Autodesk Inventor part; units mm, degrees
(part 3 of 3)
  spline S438 degree 2 poles (-141.4024, 285.9166) (-141.5043, 285.3353) (-142.1656, 284.4468) (-142.8113, 284.1243) knots 0 0 0 1 2 2 2
  spline S439 degree 2 poles (-142.8113, 284.1243) (-142.9572, 284.0514) (-143.3044, 283.9167) (-143.468, 283.8902) knots 0 0 0 1 2 2 2
  line L516 (-143.468, 283.8902) -> (-143.8192, 284.5934)
  line L517 (-143.8192, 284.5934) -> (-143.7838, 284.611)
  spline S440 degree 2 poles (-143.7838, 284.611) (-143.6644, 284.6043) (-143.2289, 284.7059) (-143.0299, 284.8053) knots 0 0 0 1 2 2 2
  spline S441 degree 2 poles (-143.0299, 284.8053) (-142.3135, 285.1631) (-141.9681, 286.5182) (-142.348, 287.4225) knots 0 0 0 1 2 2 2
  spline S442 degree 2 poles (-142.348, 287.4225) (-142.5405, 287.0777) (-142.9806, 286.6313) (-143.2945, 286.4745) knots 0 0 0 1 2 2 2
  spline S443 degree 2 poles (-143.2945, 286.4745) (-143.5952, 286.3242) (-144.1612, 286.2073) (-144.5083, 286.2715) knots 0 0 0 1 2 2 2
  spline S444 degree 2 poles (-144.5083, 286.2715) (-144.9128, 286.3513) (-145.5559, 286.8865) (-145.7967, 287.3685) knots 0 0 0 1 2 2 2
  spline S445 degree 2 poles (-142.7655, 288.3025) (-143.0416, 288.8553) (-143.5941, 289.4524) (-143.8704, 289.552) knots 0 0 0 1 2 2 2
  spline S446 degree 2 poles (-143.8704, 289.552) (-144.1179, 289.6493) (-144.5159, 289.6163) (-144.7104, 289.5191) knots 0 0 0 1 2 2 2
  spline S447 degree 2 poles (-144.7104, 289.5191) (-145.1615, 289.2938) (-145.3741, 288.3809) (-145.0692, 287.7706) knots 0 0 0 1 2 2 2
  spline S448 degree 2 poles (-145.0692, 287.7706) (-144.8969, 287.4257) (-144.4969, 287.0674) (-144.2228, 287.0054) knots 0 0 0 1 2 2 2
  spline S449 degree 2 poles (-144.2228, 287.0054) (-144.0239, 286.9611) (-143.637, 287.0604) (-143.4335, 287.162) knots 0 0 0 1 2 2 2
  spline S450 degree 2 poles (-143.4335, 287.162) (-143.1992, 287.2791) (-142.7414, 287.7122) (-142.6064, 287.9509) knots 0 0 0 1 2 2 2
  spline S451 degree 2 poles (-142.6064, 287.9509) (-142.6285, 288.0062) (-142.7103, 288.192) (-142.7655, 288.3025) knots 0 0 0 1 2 2 2
  line L518 (-359.0969, 1.8042) -> (-364.0351, 1.8396)
  line L519 (-364.0351, 1.8396) -> (-364.048, 0.0353)
  line L520 (-364.048, 0.0353) -> (-365.2097, 0.0437)
  line L521 (-365.2097, 0.0437) -> (-365.1729, 5.1845)
  line L522 (-365.1729, 5.1845) -> (-364.0112, 5.1762)
  line L523 (-364.0112, 5.1762) -> (-364.0242, 3.372)
  line L524 (-364.0242, 3.372) -> (-359.086, 3.3366)
  line L525 (-359.086, 3.3366) -> (-359.0969, 1.8042)
  line L526 (-358.9438, 10.9181) -> (-358.9795, 9.3861)
  line L527 (-358.9795, 9.3861) -> (-361.6827, 9.4489)
  line L528 (-361.6827, 9.4489) -> (-361.7311, 7.3684)
  line L529 (-361.7311, 7.3684) -> (-359.0278, 7.3055)
  line L530 (-359.0278, 7.3055) -> (-359.0634, 5.7735)
  line L531 (-359.0634, 5.7735) -> (-365.1618, 5.9153)
  line L532 (-365.1618, 5.9153) -> (-365.1262, 7.4473)
  line L533 (-365.1262, 7.4473) -> (-362.8924, 7.3954)
  line L534 (-362.8924, 7.3954) -> (-362.8441, 9.4759)
  line L535 (-362.8441, 9.4759) -> (-365.0778, 9.5278)
  line L536 (-365.0778, 9.5278) -> (-365.0422, 11.0598)
  line L537 (-365.0422, 11.0598) -> (-358.9438, 10.9181)
  line L538 (-358.8992, 12.1827) -> (-364.9945, 12.4227)
  line L539 (-364.9945, 12.4227) -> (-364.8323, 16.5422)
  line L540 (-364.8323, 16.5422) -> (-363.6715, 16.4965)
  line L541 (-363.6715, 16.4965) -> (-363.7738, 13.8984)
  line L542 (-363.7738, 13.8984) -> (-362.702, 13.8562)
  line L543 (-362.702, 13.8562) -> (-362.6076, 16.2518)
  line L544 (-362.6076, 16.2518) -> (-361.4469, 16.2061)
  line L545 (-361.4469, 16.2061) -> (-361.5412, 13.8105)
  line L546 (-361.5412, 13.8105) -> (-360.0001, 13.7498)
  line L547 (-360.0001, 13.7498) -> (-359.8978, 16.3479)
  line L548 (-359.8978, 16.3479) -> (-358.737, 16.3022)
  line L549 (-358.737, 16.3022) -> (-358.8992, 12.1827)
  line L550 (-358.1711, 26.0089) -> (-358.2682, 24.4895)
  line L551 (-358.2682, 24.4895) -> (-362.3035, 24.7473)
  line L552 (-362.3035, 24.7473) -> (-359.7694, 23.4759)
  line L553 (-359.7694, 23.4759) -> (-359.8362, 22.43)
  line L554 (-359.8362, 22.43) -> (-362.5116, 21.4914)
  line L555 (-362.5116, 21.4914) -> (-358.4762, 21.2335)
  line L556 (-358.4762, 21.2335) -> (-358.5683, 19.7931)
  line L557 (-358.5683, 19.7931) -> (-364.6558, 20.1821)
  line L558 (-364.6558, 20.1821) -> (-364.5433, 21.9432)
  line L559 (-364.5433, 21.9432) -> (-361.4526, 23.1029)
  line L560 (-361.4526, 23.1029) -> (-364.3712, 24.6368)
  line L561 (-364.3712, 24.6368) -> (-364.2586, 26.3979)
  line L562 (-364.2586, 26.3979) -> (-358.1711, 26.0089)
  line L563 (-358.069, 27.2702) -> (-364.1488, 27.7664)
  line L564 (-364.1488, 27.7664) -> (-363.8134, 31.8755)
  line L565 (-363.8134, 31.8755) -> (-362.6556, 31.781)
  line L566 (-362.6556, 31.781) -> (-362.8671, 29.1894)
  line L567 (-362.8671, 29.1894) -> (-361.798, 29.1022)
  line L568 (-361.798, 29.1022) -> (-361.6029, 31.4917)
  line L569 (-361.6029, 31.4917) -> (-360.4451, 31.3972)
  line L570 (-360.4451, 31.3972) -> (-360.6401, 29.0077)
  line L571 (-360.6401, 29.0077) -> (-359.1029, 28.8822)
  line L572 (-359.1029, 28.8822) -> (-358.8914, 31.4738)
  line L573 (-358.8914, 31.4738) -> (-357.7336, 31.3793)
  line L574 (-357.7336, 31.3793) -> (-358.069, 27.2702)
  spline S452 degree 2 poles (-357.2701, 35.0194) (-357.4024, 33.6515) (-359.2108, 32.2074) (-360.7065, 32.3521) knots 0 0 0 1 2 2 2
  spline S453 degree 2 poles (-360.7065, 32.3521) (-362.1482, 32.4915) (-363.7098, 34.2666) (-363.5775, 35.6344) knots 0 0 0 1 2 2 2
  spline S454 degree 2 poles (-363.5775, 35.6344) (-363.5427, 35.9936) (-363.4029, 36.5661) (-363.3084, 36.8251) knots 0 0 0 1 2 2 2
  spline S455 degree 2 poles (-363.3084, 36.8251) (-363.2244, 37.0256) (-362.9657, 37.4922) (-362.8722, 37.6372) knots 0 0 0 1 2 2 2
  line L575 (-362.8722, 37.6372) -> (-361.4257, 37.4972)
  line L576 (-361.4257, 37.4972) -> (-361.4404, 37.3447)
  spline S456 degree 2 poles (-361.4404, 37.3447) (-361.5498, 37.2411) (-361.8577, 36.9331) (-362.0061, 36.7339) knots 0 0 0 1 2 2 2
  spline S457 degree 2 poles (-362.0061, 36.7339) (-362.1594, 36.5352) (-362.3904, 36.046) (-362.4176, 35.7656) knots 0 0 0 1 2 2 2
  spline S458 degree 2 poles (-362.4176, 35.7656) (-362.4494, 35.4359) (-362.2956, 34.8698) (-362.0591, 34.5936) knots 0 0 0 1 2 2 2
  spline S459 degree 2 poles (-362.0591, 34.5936) (-361.8498, 34.3449) (-361.0857, 33.978) (-360.5493, 33.9261) knots 0 0 0 1 2 2 2
  spline S460 degree 2 poles (-360.5493, 33.9261) (-359.9835, 33.8714) (-359.182, 34.0968) (-358.922, 34.32) knots 0 0 0 1 2 2 2
  spline S461 degree 2 poles (-358.922, 34.32) (-358.6679, 34.5338) (-358.41, 35.0949) (-358.382, 35.3852) knots 0 0 0 1 2 2 2
  spline S462 degree 2 poles (-358.382, 35.3852) (-358.3529, 35.6853) (-358.5018, 36.251) (-358.6068, 36.4499) knots 0 0 0 1 2 2 2
  spline S463 degree 2 poles (-358.6068, 36.4499) (-358.7098, 36.6684) (-358.9406, 37.0036) (-359.033, 37.1268) knots 0 0 0 1 2 2 2
  line L577 (-359.033, 37.1268) -> (-359.0196, 37.2645)
  line L578 (-359.0196, 37.2645) -> (-357.5927, 37.1265)
  spline S464 degree 2 poles (-357.5927, 37.1265) (-357.5302, 36.9516) (-357.3757, 36.4947) (-357.3297, 36.2518) knots 0 0 0 1 2 2 2
  spline S465 degree 2 poles (-357.3297, 36.2518) (-357.2687, 35.9579) (-357.2282, 35.4524) (-357.2701, 35.0194) knots 0 0 0 1 2 2 2
  line L579 (-356.514, 43.1002) -> (-356.6871, 41.5776)
  line L580 (-356.6871, 41.5776) -> (-359.3737, 41.8829)
  line L581 (-359.3737, 41.8829) -> (-359.6087, 39.8151)
  line L582 (-359.6087, 39.8151) -> (-356.922, 39.5098)
  line L583 (-356.922, 39.5098) -> (-357.095, 37.9872)
  line L584 (-357.095, 37.9872) -> (-363.156, 38.6759)
  line L585 (-363.156, 38.6759) -> (-362.983, 40.1985)
  line L586 (-362.983, 40.1985) -> (-360.7629, 39.9462)
  line L587 (-360.7629, 39.9462) -> (-360.528, 42.014)
  line L588 (-360.528, 42.014) -> (-362.748, 42.2663)
  line L589 (-362.748, 42.2663) -> (-362.575, 43.7889)
  line L590 (-362.575, 43.7889) -> (-356.514, 43.1002)
  line L591 (-356.4432, 43.7041) -> (-362.2241, 46.5396)
  line L592 (-362.2241, 46.5396) -> (-362.0073, 48.1963)
  line L593 (-362.0073, 48.1963) -> (-355.6914, 49.4486)
  line L594 (-355.6914, 49.4486) -> (-355.896, 47.885)
  line L595 (-355.896, 47.885) -> (-357.1806, 47.6693)
  line L596 (-357.1806, 47.6693) -> (-357.4295, 45.7675)
  line L597 (-357.4295, 45.7675) -> (-356.2443, 45.2235)
  line L598 (-356.2443, 45.2235) -> (-356.4432, 43.7041)
  line L599 (-358.3221, 47.4797) -> (-360.4028, 47.1238)
  line L600 (-360.4028, 47.1238) -> (-358.4844, 46.2396)
  line L601 (-358.4844, 46.2396) -> (-358.3221, 47.4797)
  line L602 (-354.8318, 55.2679) -> (-355.0479, 53.8108)
  line L603 (-355.0479, 53.8108) -> (-359.5982, 52.1068)
  line L604 (-359.5982, 52.1068) -> (-355.393, 51.4832)
  line L605 (-355.393, 51.4832) -> (-355.5982, 50.0994)
  line L606 (-355.5982, 50.0994) -> (-361.6322, 50.9941)
  line L607 (-361.6322, 50.9941) -> (-361.3567, 52.8523)
  line L608 (-361.3567, 52.8523) -> (-357.6139, 54.2662)
  line L609 (-357.6139, 54.2662) -> (-361.071, 54.7788)
  line L610 (-361.071, 54.7788) -> (-360.8658, 56.1627)
  line L611 (-360.8658, 56.1627) -> (-354.8318, 55.2679)
  line L612 (-354.1428, 59.488) -> (-354.6718, 56.2485)
  line L613 (-354.6718, 56.2485) -> (-355.7207, 56.4198)
  line L614 (-355.7207, 56.4198) -> (-355.5797, 57.2833)
  line L615 (-355.5797, 57.2833) -> (-359.5021, 57.9238)
  line L616 (-359.5021, 57.9238) -> (-359.6431, 57.0603)
  line L617 (-359.6431, 57.0603) -> (-360.692, 57.2315)
  line L618 (-360.692, 57.2315) -> (-360.1631, 60.471)
  line L619 (-360.1631, 60.471) -> (-359.1142, 60.2997)
  line L620 (-359.1142, 60.2997) -> (-359.2552, 59.4362)
  line L621 (-359.2552, 59.4362) -> (-355.3327, 58.7957)
  line L622 (-355.3327, 58.7957) -> (-355.1917, 59.6592)
  line L623 (-355.1917, 59.6592) -> (-354.1428, 59.488)
  spline S466 degree 2 poles (-353.4, 63.0613) (-353.6397, 61.7081) (-355.5562, 60.4109) (-357.0359, 60.673) knots 0 0 0 1 2 2 2
  spline S467 degree 2 poles (-357.0359, 60.673) (-358.4621, 60.9256) (-359.879, 62.8182) (-359.6393, 64.1713) knots 0 0 0 1 2 2 2
  spline S468 degree 2 poles (-359.6393, 64.1713) (-359.5764, 64.5267) (-359.3919, 65.0864) (-359.2772, 65.3372) knots 0 0 0 1 2 2 2
  spline S469 degree 2 poles (-359.2772, 65.3372) (-359.1777, 65.5304) (-358.8831, 65.9752) (-358.7785, 66.1123) knots 0 0 0 1 2 2 2
  line L624 (-358.7785, 66.1123) -> (-357.3474, 65.8588)
  line L625 (-357.3474, 65.8588) -> (-357.3741, 65.7079)
  spline S470 degree 2 poles (-357.3741, 65.7079) (-357.4913, 65.6132) (-357.8225, 65.3305) (-357.9861, 65.1436) knots 0 0 0 1 2 2 2
  spline S471 degree 2 poles (-357.9861, 65.1436) (-358.1546, 64.9576) (-358.4235, 64.4881) (-358.4727, 64.2107) knots 0 0 0 1 2 2 2
  spline S472 degree 2 poles (-358.4727, 64.2107) (-358.5304, 63.8846) (-358.4217, 63.3081) (-358.2077, 63.0141) knots 0 0 0 1 2 2 2
  spline S473 degree 2 poles (-358.2077, 63.0141) (-358.0186, 62.7497) (-357.2858, 62.3237) (-356.7552, 62.2298) knots 0 0 0 1 2 2 2
  spline S474 degree 2 poles (-356.7552, 62.2298) (-356.1954, 62.1306) (-355.3786, 62.2922) (-355.1019, 62.4942) knots 0 0 0 1 2 2 2
  spline S475 degree 2 poles (-355.1019, 62.4942) (-354.8317, 62.6873) (-354.5304, 63.2263) (-354.4796, 63.5135) knots 0 0 0 1 2 2 2
  spline S476 degree 2 poles (-354.4796, 63.5135) (-354.427, 63.8104) (-354.5309, 64.3861) (-354.6198, 64.5926) knots 0 0 0 1 2 2 2
  spline S477 degree 2 poles (-354.6198, 64.5926) (-354.7053, 64.8186) (-354.9089, 65.1709) (-354.9913, 65.301) knots 0 0 0 1 2 2 2
  line L626 (-354.9913, 65.301) -> (-354.9672, 65.4373)
  line L627 (-354.9672, 65.4373) -> (-353.5556, 65.1873)
  spline S478 degree 2 poles (-353.5556, 65.1873) (-353.507, 65.008) (-353.3891, 64.5403) (-353.3623, 64.2946) knots 0 0 0 1 2 2 2
  spline S479 degree 2 poles (-353.3623, 64.2946) (-353.3247, 63.9967) (-353.3241, 63.4896) (-353.4, 63.0613) knots 0 0 0 1 2 2 2
  spline S480 degree 2 poles (-352.5248, 67.8341) (-352.6577, 67.1449) (-353.125, 66.1576) (-353.4052, 65.7485) knots 0 0 0 1 2 2 2
  line L628 (-353.4052, 65.7485) -> (-354.8323, 66.0237)
  line L629 (-354.8323, 66.0237) -> (-354.806, 66.1596)
  spline S481 degree 2 poles (-354.806, 66.1596) (-354.3355, 66.537) (-353.7142, 67.5399) (-353.616, 68.0495) knots 0 0 0 1 2 2 2
  spline S482 degree 2 poles (-353.616, 68.0495) (-353.5907, 68.1806) (-353.5675, 68.6141) (-353.6014, 68.7516) knots 0 0 0 1 2 2 2
  spline S483 degree 2 poles (-353.6014, 68.7516) (-353.6394, 68.92) (-353.8449, 69.1861) (-354.0439, 69.2245) knots 0 0 0 1 2 2 2
  spline S484 degree 2 poles (-354.0439, 69.2245) (-354.272, 69.2685) (-354.6218, 68.9685) (-354.7317, 68.7379) knots 0 0 0 1 2 2 2
  spline S485 degree 2 poles (-354.7317, 68.7379) (-354.8732, 68.4481) (-355.1478, 67.7811) (-355.3136, 67.4959) knots 0 0 0 1 2 2 2
  spline S486 degree 2 poles (-355.3136, 67.4959) (-355.6901, 66.8486) (-356.6362, 66.4068) (-357.2575, 66.5266) knots 0 0 0 1 2 2 2
  spline S487 degree 2 poles (-357.2575, 66.5266) (-358.0972, 66.6885) (-358.8665, 68.3119) (-358.6606, 69.3798) knots 0 0 0 1 2 2 2
  spline S488 degree 2 poles (-358.6606, 69.3798) (-358.5577, 69.9137) (-358.1352, 70.9297) (-357.8703, 71.3116) knots 0 0 0 1 2 2 2
  line L630 (-357.8703, 71.3116) -> (-356.5015, 71.0476)
  line L631 (-356.5015, 71.0476) -> (-356.5268, 70.9166)
  spline S489 degree 2 poles (-356.5268, 70.9166) (-356.8777, 70.6369) (-357.4562, 69.7516) (-357.5535, 69.2468) knots 0 0 0 1 2 2 2
  spline S490 degree 2 poles (-357.5535, 69.2468) (-357.5919, 69.0478) (-357.5936, 68.7259) (-357.5496, 68.5362) knots 0 0 0 1 2 2 2
  spline S491 degree 2 poles (-357.5496, 68.5362) (-357.5136, 68.3833) (-357.3006, 68.1308) (-357.1452, 68.1008) knots 0 0 0 1 2 2 2
  spline S492 degree 2 poles (-357.1452, 68.1008) (-356.9122, 68.0559) (-356.5826, 68.3296) (-356.3859, 68.775) knots 0 0 0 1 2 2 2
  spline S493 degree 2 poles (-356.3859, 68.775) (-356.2599, 69.0628) (-356.0213, 69.5957) (-355.8478, 69.8946) knots 0 0 0 1 2 2 2
  spline S494 degree 2 poles (-355.8478, 69.8946) (-355.4999, 70.4719) (-354.6257, 70.9326) (-354.0044, 70.8128) knots 0 0 0 1 2 2 2
  spline S495 degree 2 poles (-354.0044, 70.8128) (-353.1113, 70.6406) (-352.2945, 69.0281) (-352.5248, 67.8341) knots 0 0 0 1 2 2 2
  constraints: 2 centre point, 2 coincident, 2 other
extrude "Extrusion11" cut sketch "Sketch11" against normal blind 1 contours L320 L321 L322 S221 S222 S219 S220 | L0 L1 L2 S2 S3 S0 S1 | L510 L511 L512 L513 L514 L515 L509 | L6 L7 L8 L9 L10 L11 L12 L13 L14 L15 L16 L17 | L36 L25 L26 L27 L28 L29 L30 L31 L32 L33 L34 L35 | L103 L104 L105 L106 L107 L108 L109 L116 | L124 L125 L126 L127 L128 L129 L130 L131 L120 L121 L122 L123 | L150 L151 S119 S120 S121 S122 S123 S124 L152 L153 S125 S126 S127 S128 S129 L154 L155 | L156 L157 L158 L159 L160 L161 S130 L162 L163 L164 L165 | L168 L169 L170 S152 S153 S150 S151 | L250 L251 L252 L253 L254 L255 L256 L257 L258 L246 L247 L248 L249 | L352 L353 S281 S282 S283 S284 S285 S286 L354 L355 S287 S288 S289 S290 S291 L356 L357 | L399 L388 L389 L390 L391 L392 L393 L394 L395 L396 L397 L398 | L400 L401 L402 L403 L404 L405 | L433 L422 L423 L424 L425 L426 L427 L428 L429 L430 L431 L432 | L440 L441 L442 L443 L434 L435 L436 L437 L438 L439 | L477 L478 L479 S373 S374 S371 S372 | S379 L495 L496 S380 S381 S382 S383 S384 S385 S386 S387 L497 L498 S388 S389 S390 S391 S392 S393 S394 A1 | A1 S394 S379 | A1 L414 L415 L416 L417 L418 L419 L420 | S397 S398 S399 S400 S401 L499 L500 S402 S403 S404 S405 S406 S395 S396 A1 | A1 S396 S397 | S370 S355 A1 | A1 S355 L410 L411 S356 S357 S358 S359 S360 S361 S362 S363 L412 L413 S364 S365 S366 S367 S368 S369 S370 | S424 L504 L505 S425 S426 S427 S428 S429 L506 L507 L508 S430 S431 S432 S414 S415 L501 L502 S416 S417 S418 S419 L503 S420 S421 S422 S423 A1 | A1 S423 S424 | S354 S339 A1 | A1 S339 L406 L407 S340 S341 S342 S343 S344 S345 S346 S347 L408 L409 S348 S349 S350 S351 S352 S353 S354 | L516 L517 S440 S441 S442 S443 S444 S433 S434 S435 S436 S437 S438 A1 | A1 S438 S439 L516 | S327 S328 A1 | A1 S328 S329 S330 S331 S332 S325 S326 S327 | S324 S311 A1 | A1 S311 S312 S313 S314 S315 S316 L381 L382 S317 S318 S319 S320 S321 S322 L383 L384 L385 L386 L387 S323 S324 | S11 S12 S13 S14 S15 S8 S9 S10 A1 | A1 S10 S11 | S300 S292 A1 | A1 S292 S293 S294 L358 S295 S296 S297 S298 L359 S299 S300 | S22 S23 S24 S25 S26 S27 L18 L19 S28 S29 S30 S31 S32 S33 L20 L21 L22 L23 L24 S34 S35 A1 | A1 S35 S22 | S271 S272 A1 | A1 S272 L347 L348 S273 S274 S275 S276 S277 L349 L350 L351 S278 S279 S280 S262 S263 L344 L345 S264 S265 S266 S267 L346 S268 S269 S270 S271 | S36 L59 L60 S37 S38 S39 S40 S41 S42 S43 S44 L61 L62 S45 S46 S47 S48 S49 S50 S51 A1 | A1 S51 S36 | S244 S245 A1 | A1 S245 S246 S247 S248 S249 L342 L343 S250 S251 S252 S253 S254 S243 S244 | L63 L64 L65 L66 L67 L68 L69 A1 | S242 S227 A1 | A1 S227 L338 L339 S228 S229 S230 S231 S232 S233 S234 S235 L340 L341 S236 S237 S238 S239 S240 S241 S242 | S52 L71 L72 S53 S54 S55 S56 S57 S58 S59 S60 L73 L74 S61 S62 S63 S64 S65 S66 S67 A1 | A1 S67 S52 | S68 S69 S70 S71 S72 S73 L87 L88 S74 S75 S76 S77 S78 S79 S80 S81 L89 L90 S82 S83 A1 | A1 S83 S68 | S218 S211 A1 | A1 S211 S212 L292 L293 L294 S213 S214 S215 S216 L295 L296 L297 S217 S218 | S199 S200 A1 | A1 S200 S201 S202 S203 S204 S197 S198 S199 | S84 L144 L145 S85 S86 S87 S88 S89 S90 S91 S92 L146 L147 S93 S94 S95 S96 S97 S98 S99 A1 | A1 S99 S84 | L116 L109 L108 | L108 L109 L110 L111 L112 L113 L114 L115 L116 | S196 S181 A1 | A1 S181 L277 L278 S182 S183 S184 S185 S186 S187 S188 S189 L279 L280 S190 S191 S192 S193 S194 S195 S196 | S102 S103 S104 S105 S106 L148 L149 S107 S108 S109 S110 S111 S100 S101 A1 | A1 S101 S102 | A1 L269 L270 L271 L272 L273 L274 L275 | S180 S165 A1 | A1 S165 L242 L243 S166 S167 S168 S169 S170 S171 S172 S173 L244 L245 S174 S175 S176 S177 S178 S179 S180 | S133 S134 S135 S136 S137 L166 L167 S138 S139 S140 S141 S142 S131 S132 A1 | A1 S132 S133 | A1 L211 L212 L213 L214 L215 L216 L217 | L258 L257 L246 | L257 L258 L259 L260 L261 L262 L263 L264 L265 | L612 L613 L614 L615 L616 L617 L618 L619 L620 L621 L622 L623 | L549 L538 L539 L540 L541 L542 L543 L544 L545 L546 L547 L548 | L574 L563 L564 L565 L566 L567 L568 L569 L570 L571 L572 L573 | L603 L604 L605 L606 L607 L608 L609 L610 L611 L602 | L580 L581 L582 L583 L584 L585 L586 L587 L588 L589 L590 L579 | S466 S467 S468 S469 L624 L625 S470 S471 S472 S473 S474 S475 S476 S477 L626 L627 S478 S479 A2 | A2 S479 S466 | S465 S452 A2 | A2 S452 S453 S454 S455 L575 L576 S456 S457 S458 S459 S460 S461 S462 S463 L577 L578 S464 S465 | S480 L628 L629 S481 S482 S483 S484 S485 S486 S487 S488 L630 L631 S489 S490 S491 S492 S493 S494 S495 A2 | A2 S495 S480 | L527 L528 L529 L530 L531 L532 L533 L534 L535 L536 L537 L526 | L518 L519 L520 L521 L522 L523 L524 A2 | L37 L38 L39 L40 L41 L42 L43 L44 L45 L46 | L47 L48 L49 L50 L51 L52 L53 L54 L55 L56 L57 L58 | L75 L76 L77 L78 L79 L80 L81 L82 L83 L84 L85 L86 | L91 L92 L93 L94 L95 L96 L97 L98 L99 L100 L101 L102 | L132 L133 L134 L135 L136 L137 L138 L139 L140 L141 L142 L143 | L174 L175 L176 L177 L178 L179 L180 L181 L182 L183 L184 L185 | L186 L187 L188 L189 L190 L191 L192 L193 L194 L195 L196 L197 L198 | L199 L200 L201 L202 L203 L204 L205 L206 L207 L208 L209 L210 | L219 L220 L221 L222 L223 L224 L225 S158 S159 S160 L226 | L230 L231 L232 L233 L234 L235 L236 L237 L238 L239 L240 L241 | L281 L282 L283 L284 L285 L286 L287 L288 | L298 L299 L300 L301 L302 L303 L304 L305 L306 L307 | L308 L309 L310 L311 L312 L313 L314 L315 L316 L317 L318 L319 | L326 L327 L328 L329 L330 L331 L332 L333 L334 L335 L336 L337 | L360 L361 L362 L363 L364 L365 L366 L367 | L371 L372 L373 L374 L375 L376 L377 L378 L379 L380 | L444 L445 L446 L447 L448 L449 L450 L451 | L455 L456 L457 L458 L459 L460 L461 L462 L463 L464 | L465 L466 L467 L468 L469 L470 L471 L472 L473 L474 L475 L476 | L483 L484 L485 L486 L487 L488 L489 L490 L491 L492 L493 L494 | L550 L551 L552 L553 L554 L555 L556 L557 L558 L559 L560 L561 L562 | L591 L592 L593 L594 L595 L596 L597 L598
body "Solid2"
